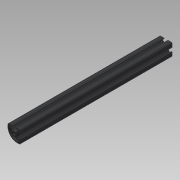
# Autodesk Inventor part: 1012
Saved by Autodesk Inventor 2013 (Build 170138000, 138)
## iProperties
Company: 80/20 Inc.
Created: 2013-09-06
Part Number: 1012
Material: Generic
Document SubType Name: Modeling
Density: 1 g/cm^3
Catalog Web Link: 8020.net
Vendor: 80/20 Inc.
Engineer: Ross Bowman
Author: Ross Bowman
Keywords: T-Slot, Extrusion, 80/20, 8020, Quick Frame, HT
Autodesk Inventor part; units mm, degrees
ref_plane "YZ Plane" through (0, 0, 0) normal (1, 0, 0) x (0, 1, 0)
ref_plane "XZ Plane" through (0, 0, 0) normal (0, 1, 0) x (-1, 0, 0)
ref_plane "XY Plane" through (0, 0, 0) normal (0, 0, 1) x (1, 0, 0)
sketch "Sketch1" plane through (0, 0, 0) normal (0, 0, 1) x (1, 0, 0)
  arc A0 (-11.5663, -0.1236) -> (-11.886, 0.8407) centre (-11.7326, 0.3564) ccw
  arc A1 (-11.5663, -0.1236) -> (-10.4403, -2.6494) centre (6.35, 6.35) ccw
  arc A2 (-12.7, 6.35) -> (-11.886, 0.8407) centre (6.35, 6.35) ccw
  arc A3 (-9.9367, -3.5317) -> (-10.4403, -2.6494) centre (-10.1943, -3.0939) ccw
  line L0 (-12.7, 6.35) -> (-12.7, 9.5504)
  arc A4 (-9.9367, -3.5317) -> (-3.5317, -9.9367) centre (6.35, 6.35) ccw
  arc A5 (-12.7, 9.5504) -> (-12.7, 10.5664) centre (-12.7, 10.0584) ccw
  arc A6 (-2.6494, -10.4403) -> (-3.5317, -9.9367) centre (-3.0939, -10.1943) ccw
  line L1 (-12.7, 10.5664) -> (-12.7, 10.5918)
  arc A7 (-2.6494, -10.4403) -> (-0.1348, -11.5623) centre (6.35, 6.35) ccw
  arc A8 (-10.5918, 12.7) -> (-12.7, 10.5918) centre (-10.5918, 10.5918) ccw
  arc A9 (0.8294, -11.8825) -> (-0.1348, -11.5623) centre (0.3459, -11.7266) ccw
  line L2 (-10.5918, 12.7) -> (-10.5664, 12.7)
  arc A10 (0.8294, -11.8825) -> (6.35, -12.7) centre (6.35, 6.35) ccw
  arc A11 (-10.5664, 12.7) -> (-9.5504, 12.7) centre (-10.0584, 12.7) ccw
  line L3 (9.5504, -12.7) -> (6.35, -12.7)
  line L4 (-9.5504, 12.7) -> (-6.3246, 12.7)
  arc A12 (10.5664, -12.7) -> (9.5504, -12.7) centre (10.0584, -12.7) ccw
  arc A13 (-6.3246, 12.7) -> (-5.3086, 12.7) centre (-5.8166, 12.7) ccw
  line L5 (10.5918, -12.7) -> (10.5664, -12.7)
  line L6 (-5.3086, 12.7) -> (-4.3561, 12.7)
  arc A14 (10.5918, -12.7) -> (12.7, -10.5918) centre (10.5918, -10.5918) ccw
  arc A15 (-4.3561, 10.4902) -> (-4.3561, 12.7) centre (-4.3561, 11.5951) ccw
  line L7 (12.7, -10.5664) -> (12.7, -10.5918)
  line L8 (-4.3561, 10.4902) -> (-6.4748, 10.4902)
  arc A16 (12.7, -9.5504) -> (12.7, -10.5664) centre (12.7, -10.0584) ccw
  arc A17 (-6.4748, 10.4902) -> (-7.1932, 8.7558) centre (-6.4748, 9.4742) ccw
  line L9 (12.7, -6.3246) -> (12.7, -9.5504)
  line L10 (-7.1932, 8.7558) -> (-3.8759, 5.4384)
  arc A18 (12.7, -5.3086) -> (12.7, -6.3246) centre (12.7, -5.8166) ccw
  arc A19 (-3.8759, 5.4384) -> (-1.6308, 4.5085) centre (-1.6308, 7.6835) ccw
  line L11 (12.7, -4.3561) -> (12.7, -5.3086)
  line L12 (-1.6308, 4.5085) -> (1.6308, 4.5085)
  arc A20 (12.7, -4.3561) -> (10.4902, -4.3561) centre (11.5951, -4.3561) ccw
  arc A21 (1.6308, 4.5085) -> (3.8759, 5.4384) centre (1.6308, 7.6835) ccw
  line L13 (10.4902, -6.4748) -> (10.4902, -4.3561)
  line L14 (7.1932, 8.7558) -> (3.8759, 5.4384)
  arc A22 (8.7558, -7.1932) -> (10.4902, -6.4748) centre (9.4742, -6.4748) ccw
  arc A23 (7.1932, 8.7558) -> (6.4748, 10.4902) centre (6.4748, 9.4742) ccw
  line L15 (8.7558, -7.1932) -> (5.4384, -3.8759)
  line L16 (6.4748, 10.4902) -> (4.3561, 10.4902)
  arc A24 (4.5085, -1.6308) -> (5.4384, -3.8759) centre (7.6835, -1.6308) ccw
  arc A25 (4.3561, 12.7) -> (4.3561, 10.4902) centre (4.3561, 11.5951) ccw
  line L17 (4.5085, 1.6308) -> (4.5085, -1.6308)
  line L18 (4.3561, 12.7) -> (5.3086, 12.7)
  arc A26 (5.4384, 3.8759) -> (4.5085, 1.6308) centre (7.6835, 1.6308) ccw
  arc A27 (5.3086, 12.7) -> (6.3246, 12.7) centre (5.8166, 12.7) ccw
  line L19 (8.7558, 7.1932) -> (5.4384, 3.8759)
  line L20 (6.3246, 12.7) -> (9.5504, 12.7)
  arc A28 (10.4902, 6.4748) -> (8.7558, 7.1932) centre (9.4742, 6.4748) ccw
  arc A29 (9.5504, 12.7) -> (10.5664, 12.7) centre (10.0584, 12.7) ccw
  line L21 (10.4902, 4.3561) -> (10.4902, 6.4748)
  line L22 (10.5664, 12.7) -> (10.5918, 12.7)
  arc A30 (10.4902, 4.3561) -> (12.7, 4.3561) centre (11.5951, 4.3561) ccw
  arc A31 (12.7, 10.5918) -> (10.5918, 12.7) centre (10.5918, 10.5918) ccw
  line L23 (12.7, 5.3086) -> (12.7, 4.3561)
  line L24 (12.7, 10.5918) -> (12.7, 10.5664)
  arc A32 (12.7, 6.3246) -> (12.7, 5.3086) centre (12.7, 5.8166) ccw
  arc A33 (12.7, 10.5664) -> (12.7, 9.5504) centre (12.7, 10.0584) ccw
  line L25 (12.7, 9.5504) -> (12.7, 6.3246)
  arc A34 (-4.5085, 0.2413) -> (0.2413, -4.5085) centre (0.2413, 0.2413) ccw
  line L26 (0.2413, -4.5085) -> (1.6308, -4.5085)
  line L27 (-4.5085, 1.6308) -> (-4.5085, 0.2413)
  arc A35 (3.8759, -5.4384) -> (1.6308, -4.5085) centre (1.6308, -7.6835) ccw
  arc A36 (-4.5085, 1.6308) -> (-5.4384, 3.8759) centre (-7.6835, 1.6308) ccw
  line L28 (3.8759, -5.4384) -> (7.1927, -8.7553)
  line L29 (-8.7553, 7.1927) -> (-5.4384, 3.8759)
  arc A37 (6.4823, -10.4897) -> (7.1927, -8.7553) centre (6.4743, -9.4737) ccw
  arc A38 (-8.7553, 7.1927) -> (-10.4897, 6.4823) centre (-9.4737, 6.4743) ccw
  arc A39 (-10.4897, 6.4823) -> (6.4823, -10.4897) centre (6.35, 6.35) ccw
  circle A40 centre (0, 0) radius 2.6035
  constraints: 80 point on circle, 60 end point, 41 centre point
extrude "Extrusion1" add sketch "Sketch1" against normal blind 304.8
body "Solid1"
